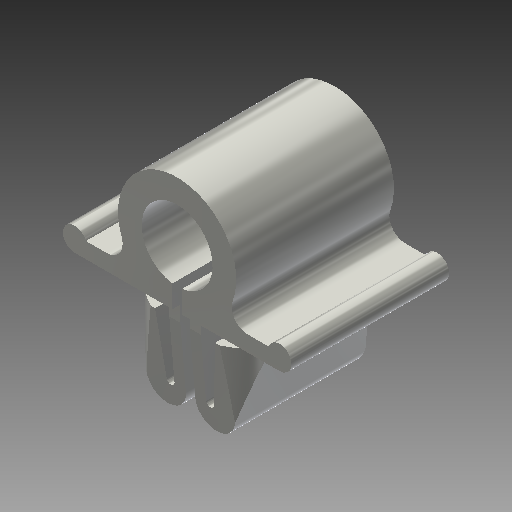
# Autodesk Inventor part: 202-15
Saved by Autodesk Inventor 2019 (Build 230136000, 136)
## iProperties
Company: Autodesk Inc.
Created: 2007-11-04
Part Number: 202-15
Document SubType Name: Modeling
Designer: Autodesk Inc.
Density: 1.06 g/cm^3
Mass: 0.651674 g
Surface Area: 10.936 cm^2
Volume: 0.614787 cm^3
Material: ABS Plastic
Description: WIRE CLIP
Appearance: Smooth - Ivory
Component Category: Fasteners
Author: Inventor
Autodesk Inventor part; units mm, degrees
ref_plane "YZ Plane" through (0, 0, 0) normal (1, 0, 0) x (0, 1, 0)
ref_plane "XZ Plane" through (0, 0, 0) normal (0, 1, 0) x (-1, 0, 0)
ref_plane "XY Plane" through (0, 0, 0) normal (0, 0, 1) x (1, 0, 0)
sketch "Sketch1" plane through (0, 0, 0) normal (0, 0, 1) x (1, 0, 0)
  circle A0 centre (0, 0) radius 2.25
  arc A1 (-5.7929, -2.643) -> (-6.5, -3.643) centre (-6.5, -2.893) ccw
  arc A2 (6.5, -3.643) -> (5.7929, -2.643) centre (6.5, -2.893) ccw
  line L0 (-5.7929, -2.643) -> (-4.4568, -2.643)
  line L1 (5.7929, -2.643) -> (4.4568, -2.643)
  arc A3 (3.5185, -1.2971) -> (-3.5185, -1.2971) centre (0, 0) ccw
  arc A4 (-4.4568, -2.643) -> (-3.5185, -1.2971) centre (-4.4568, -1.643) ccw
  arc A5 (3.5185, -1.2971) -> (4.4568, -2.643) centre (4.4568, -1.643) ccw
  line L2 (-0.3, -2.2299) -> (-0.3, -8.643)
  line L3 (0.3, -2.2299) -> (0.3, -3.643)
  arc A6 (-2.7514, -8.9882) -> (-0.3, -8.643) centre (-1.55, -8.643) ccw
  line L4 (-2.7514, -8.9882) -> (-4, -4.643)
  line L5 (-4, -4.643) -> (-1.9, -4.643)
  arc A7 (-1.4986, -8.4691) -> (-1, -8.443) centre (-1.25, -8.443) ccw
  line L6 (-1.9, -4.643) -> (-1.4986, -8.4691)
  line L7 (-1, -3.643) -> (-1, -8.443)
  line L8 (-12.8733, -3.643) -> (-1, -3.643)
  line L9 (1, -3.643) -> (16.2885, -3.643)
  line L10 (0, 6.5107) -> (0, -12.8141) projected
  line L11 (0.3, -2.2299) -> (0.3, -8.643)
  arc A8 (0.3, -8.643) -> (2.7514, -8.9882) centre (1.55, -8.643) ccw
  line L12 (2.7514, -8.9882) -> (4, -4.643)
  line L13 (4, -4.643) -> (1.9, -4.643)
  arc A9 (1, -8.443) -> (1.4986, -8.4691) centre (1.25, -8.443) ccw
  line L14 (1.9, -4.643) -> (1.4986, -8.4691)
  line L15 (1, -3.643) -> (1, -8.443)
  dimension "d0" = 4.5
  dimension "d5" = 1.5
  dimension "d6" = 1.5
  dimension "d7" = 6.5
  dimension "d8" = 6.5
  dimension "d9" = 3.75
  dimension "d10" = 1
  dimension "d11" = 0.6
  dimension "d12" = 0.3
  dimension "d13" = 0.5
  dimension "d14" = 2.5
  dimension "d15" = 4
  dimension "d17" = 2.1
  dimension "d18" = 0.2
  dimension "d19" = 0.7
  dimension "d21" = 3.643
  dimension "d22" = 1
  dimension "d23" = 1
  dimension "d24" = 5
  dimension "d25" = 1
  constraints: 30 end point, 20 point on circle, 12 tangent, 10 centre point, 9 symmetric about line, 3 parallel, 3 perpendicular, 2 coincident, 2 horizontal, 2 point on line, 1 collinear, 1 equal radius, 2 other
  measures "d0" diameter of A0
  measures "d5" diameter of A1
  measures "d6" diameter of A2
  measures "d7" horizontal distance of point (0, 0) A1.centre
  measures "d8" horizontal distance of point (0, 0) A2.centre
  measures "d9" radius of A3
  measures "d10" radius of A4
  measures "d11" distance between parallel lines of L2 L3
  measures "d12" distance from line of point (0, 0) L2
  measures "d13" diameter of A7
  measures "d14" diameter of A6
  measures "d15" horizontal distance of point (0, 0) L4.end
  measures "d17" distance of L4.end L5.end
  measures "d18" vertical distance of A6.centre A7.centre
  measures "d19" distance between parallel lines of L7 L2
  measures "d21" distance from line of point (0, 0) L8
  measures "d22" distance between parallel lines of L8 L0
  measures "d23" distance between parallel lines of L9 L1
  measures "d24" distance from line of L8 A6.centre
  measures "d25" distance between parallel lines of L8 L5
extrude "Extrusion1" add sketch "Sketch1" along normal mid plane 10 contours A0 L10 A3 A5 L1 A2 L9 L15 A9 L14 L13 L12 A8 L11 L3 | A0 L2 A6 L4 L5 L6 A7 L7 L8 A1 L0 A4 A3 L10
sketch "Sketch2" plane through (1, -3.643, 5) normal (0, -1, 0) x (1, 0, 0)
  circle A0 centre (-1, -5) radius 10
  circle A1 centre (-1, -5) radius 5
  dimension "d28" = 10
  dimension "d29" = 5
  constraints: 2 centre point, 2 coincident
  measures "d28" diameter of A1
  measures "d29" radial gap between concentric circles of A1 A0
extrude "Extrusion2" cut sketch "Sketch2" along normal through all
sketch "Sketch3" plane through (0, 0, 0) normal (1, 0, 0) x (0, 1, 0)
  line L0 (-3.643, 5) -> (-3.643, 4.991) projected
  line L1 (-3.643, -5) -> (-3.643, 5) projected
  line L2 (-3.643, -4.991) -> (-3.643, -5) projected
  line L3 (-3.643, -4.899) -> (-3.643, -4.991) projected
  line L4 (-3.643, -4.899) -> (-3.643, 4.899) projected
  line L5 (-3.643, 4.991) -> (-3.643, 4.899) projected
  line L6 (-3.643, 5) -> (-3.643, 4.5)
  line L7 (-11.643, 3.8876) -> (-11.643, 6)
  line L8 (-11.643, 6) -> (-3.643, 6)
  line L9 (-3.643, 6) -> (-3.643, 5)
  line L10 (-3.643, 4.5) -> (-4.643, 4.5)
  line L11 (-4.643, 4.5) -> (-11.643, 3.8876)
  line L12 (-13.9716, 0) -> (2.3286, 0) projected
  line L13 (-3.643, -5) -> (-3.643, -4.991)
  line L14 (-3.643, -4.991) -> (-3.643, -4.899)
  line L15 (-3.643, -5) -> (-3.643, -4.5)
  line L16 (-11.643, -3.8876) -> (-11.643, -6)
  line L17 (-11.643, -6) -> (-3.643, -6)
  line L18 (-3.643, -6) -> (-3.643, -5)
  line L19 (-3.643, -4.5) -> (-4.643, -4.5)
  line L20 (-4.643, -4.5) -> (-11.643, -3.8876)
  point P0 (0, 0)
  dimension "d32" = 1
  dimension "d33" = 5
  dimension "d34" = 0.5
  dimension "d35" = 1
  dimension "d36" = 8
  constraints: 28 end point, 7 symmetric about line, 2 perpendicular, 1 collinear, 1 parallel, 1 point on line
  measures "d32" distance of L6.end L10.end
  measures "d33" angle of L10 L11
  measures "d34" distance from line of L10 L0.start
  measures "d35" distance of L8.end L1.end
  measures "d36" distance of L7.end L8.end
extrude "Extrusion3" cut sketch "Sketch3" along normal through all both and the other way through all
equation "\"d6\" = d5"
equation "\"d8\" = d7"
equation "\"d12\" = 0.5 * d11"
equation "\"d4\" = d3"
equation "\"d3\" = 1"
body "Solid1"
